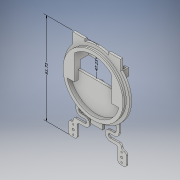
# Autodesk Inventor part: vivetouchpad
Saved by Autodesk Inventor 2019.4 (Build 234330000, 330)
## iProperties
Created: 2021-01-30
Part Number: vivetouchpad
Material: Generic
Document SubType Name: Modeling
Designer: Ian
Density: 1 g/cm^3
Appearance: Default
Author: Ian
Autodesk Inventor part; units mm, degrees
ref_plane "YZ Plane" through (0, 0, 0) normal (1, 0, 0) x (0, 1, 0)
ref_plane "XZ Plane" through (0, 0, 0) normal (0, 1, 0) x (-1, 0, 0)
ref_plane "XY Plane" through (0, 0, 0) normal (0, 0, 1) x (1, 0, 0)
sketch "Sketch1" plane through (0, 0, 0) normal (0, 0, 1) x (1, 0, 0)
  circle A0 centre (0, 0) radius 22
  line L0 (-4, -21.6333) -> (-4, -25.1333)
  line L1 (-4, -25.1333) -> (4, -25.1333)
  line L2 (4, -25.1333) -> (4, -21.6333)
  line L3 (-16, 15.0997) -> (-16, 22.0997)
  line L4 (-16, 22.0997) -> (-8, 22.0997)
  line L5 (-8, 22.0997) -> (-8, 20.4939)
  line L6 (8, 20.4939) -> (8, 22.0997)
  line L7 (8, 22.0997) -> (16, 22.0997)
  line L8 (16, 22.0997) -> (16, 15.0997)
  circle A1 centre (0, 0) radius 2.75
  circle A2 centre (0, 0) radius 1.25 construction
  circle A3 centre (0, 0) radius 1.35
  dimension "d0" = 44
  dimension "d1" = 8
  dimension "d2" = 16
  dimension "d3" = 7
  dimension "d4" = 8
  dimension "d5" = 3.5
  dimension "d6" = 2.5
  dimension "d7" = 0.1
  dimension "d8" = 5.5
  constraints: 18 end point, 6 point on circle, 5 perpendicular, 4 centre point, 4 parallel, 3 coincident, 2 point on line, 2 vertical
  measures "d0" diameter of A0
  measures "d1" distance of L6.end L7.end
  measures "d2" distance between parallel lines of L6 L5
  measures "d3" distance of L7.end L8.end
  measures "d4" distance of L0.end L1.end
  measures "d5" distance of L1.end L2.end
  measures "d6" diameter of A2
  measures "d7" radial gap between concentric circles of A2 A3
  measures "d8" diameter of A1
extrude "Extrusion1" add sketch "Sketch1" along normal blind 1.5 contours A0 | A0 L6 L7 L8 | L2 L1 L0 A0 | A0 L3 L4 L5 | A1 | A3
sketch "Sketch10" plane through (0, 0, 0) normal (0, 0, -1) x (-1, 0, 0)
  circle A0 centre (0, -1.6753) radius 1.25 construction
  circle A1 centre (0, -1.6753) radius 2.625
  line L0 (-16, 22.0997) -> (-8, 22.0997) construction
  point P0 (0, 0)
  dimension "d85" = 5.25
  dimension "d86" = 2.5
  dimension "d87" = 26.4
  constraints: 2 centre point, 1 coincident, 1 vertical alignment
  measures "d85" diameter of A1
  measures "d86" diameter of A0
extrude "Extrusion8" add sketch "Sketch10" along normal blind 2.3
sketch "Sketch11" plane through (0, -1.6753, -2.3) normal (0, 0, -1) x (-1, 0, 0)
  circle A0 centre (0, 0) radius 1.25 construction
  circle A1 centre (0, 0) radius 1.35
  circle A2 centre (0, 0) radius 1.65
  point P0 (0, 1.6753)
  dimension "d90" = 2.5
  dimension "d91" = 0.1
  dimension "d92" = 0.3
  constraints: 3 centre point
  measures "d90" diameter of A0
  measures "d91" radial gap between concentric circles of A0 A1
  measures "d92" radial gap between concentric circles of A1 A2
extrude "Extrusion9" add sketch "Sketch11" along normal blind 0.2
chamfer "Chamfer1" distance 0.975 angle 45 1 edges at (2.625, -1.6753, -2.3)
fillet "Fillet1" radius 2 1 edges at (2.625, -1.6753, -1.3251)
fillet "Fillet2" radius 0.5 2 edges at (1.6501, -1.6753, -2.3) (1.65, -1.6753, -2.3)
sketch "Sketch8" plane through (0, 0, 1.5) normal (0, 0, 1) x (1, 0, 0)
  circle A0 centre (0, 0) radius 1.35 projected
  circle A1 centre (0, 0) radius 19.875
  circle A2 centre (0, 0) radius 17.875
  dimension "d78" = 39.75
  dimension "d79" = 2
  constraints: 2 centre point, 1 coincident
  measures "d78" diameter of A1
  measures "d79" radial gap between concentric circles of A1 A2
extrude "Extrusion6" add sketch "Sketch8" along normal blind 2.5 contours A1
sketch "Sketch9" plane through (0, 0, 4) normal (0, 0, 1) x (1, 0, 0)
  circle A0 centre (0, 0) radius 17.875 projected
  circle A1 centre (0, 0) radius 19.875 projected
  circle A2 centre (0, 0) radius 20.15
  dimension "d82" = 40.3
  constraints: 1 centre point, 1 coincident
  measures "d82" diameter of A2
extrude "Extrusion7" add sketch "Sketch9" against normal blind 1 contours A1 | A2
sketch "Sketch12" plane through (0, 0, 0) normal (0, 0, -1) x (-1, 0, 0)
  line L0 (-12.5, 1.875) -> (12.5, 1.875)
  circle A0 centre (0, 0) radius 17.875 construction
  circle A1 centre (0, -1.6753) radius 2.625 construction
  arc A2 (12.5, 12.7775) -> (-12.5, 12.7775) centre (0, 0) ccw
  line L1 (-12.5, 12.7775) -> (-12.5, 1.875)
  line L2 (12.5, 1.875) -> (12.5, 12.7775)
  dimension "d100" = 25
  dimension "d101" = 16
  dimension "d102" = 6.1753
  constraints: 6 end point, 4 point on circle, 2 concentric, 2 parallel, 1 centre point, 1 horizontal, 1 vertical
  measures "d100" distance of L0.start L0.end
  measures "d101" distance edge to line of A0 L0
extrude "Extrusion10" cut sketch "Sketch12" against normal through all
sketch "Sketch6" plane through (0, 0, 0) normal (0, 0, -1) x (-1, 0, 0)
  arc A0 (8.5, -23.1333) -> (8.5, -29.6333) centre (8.5, -26.3833) ccw
  arc A1 (8.5, -25.1333) -> (8.5, -27.6333) centre (8.5, -26.3833) ccw
  line L0 (4, -25.1333) -> (-4, -25.1333) construction
  line L1 (-4, -25.1333) -> (29.2645, -25.1333) construction
  line L2 (0, -1.6753) -> (0, -71.0097) construction
  line L3 (8.5, -26.3833) -> (8.5, -20.6854) construction
  arc A2 (4, -21.6333) -> (16, 15.0997) centre (0, 0) ccw construction
  line L4 (16, 22.0997) -> (16, 15.0997) projected
  line L5 (8, 22.0997) -> (16, 22.0997) projected
  line L6 (8, 20.4939) -> (8, 22.0997) projected
  arc A3 (8, 20.4939) -> (-8, 20.4939) centre (0, 0) ccw projected
  line L7 (-8, 22.0997) -> (-8, 20.4939) projected
  line L8 (-16, 22.0997) -> (-8, 22.0997) projected
  line L9 (-16, 15.0997) -> (-16, 22.0997) projected
  arc A4 (-16, 15.0997) -> (-4, -21.6333) centre (0, 0) ccw projected
  line L10 (-4, -25.1333) -> (-4, -21.6333) projected
  line L11 (4, -25.1333) -> (-4, -25.1333) projected
  line L12 (4, -21.6333) -> (4, -25.1333) projected
  arc A5 (4, -21.6333) -> (16, 15.0997) centre (0, 0) ccw projected
  line L13 (8.5, -27.6333) -> (14.5, -27.6333)
  line L14 (8.5, -29.6333) -> (12.0333, -29.6333)
  line L15 (19.5, -32.6333) -> (19.5, -37.9666)
  line L16 (17.8333, -39.6333) -> (15.3667, -39.6333)
  line L17 (17.8333, -39.6333) -> (13.7, -39.6333)
  line L18 (13.7, -37.9666) -> (13.7, -32.6333)
  line L19 (13.7, -32.6333) -> (19.5, -32.6333) construction
  line L20 (19.5, -32.6333) -> (19.5, -37.9666)
  circle A6 centre (16.25, -32.1333) radius 0.5
  circle A7 centre (16.25, -38.1333) radius 0.5
  circle A8 centre (16.25, -35.1333) radius 0.75
  line L21 (16.25, -35.1333) -> (16.25, -32.1333) construction
  line L22 (16.25, -35.1333) -> (16.25, -38.1333) construction
  arc A9 (19.5, -32.6333) -> (17.8333, -30.9666) centre (17.8333, -32.6333) ccw
  arc A10 (16.1667, -29.3) -> (17.8333, -30.9666) centre (17.8333, -29.3) ccw
  arc A11 (16.1667, -29.3) -> (14.5, -27.6333) centre (14.5, -29.3) ccw
  arc A12 (13.7, -31.3) -> (12.0333, -29.6333) centre (12.0333, -31.3) ccw
  line L23 (13.7, -32.6333) -> (13.7, -31.3)
  arc A13 (17.8333, -39.6333) -> (19.5, -37.9666) centre (17.8333, -37.9666) ccw
  arc A14 (13.7, -37.9666) -> (15.3667, -39.6333) centre (15.3667, -37.9666) ccw
  arc A15 (4, -21.6333) -> (16, 15.0997) centre (0, 0) ccw projected
  line L24 (16, 22.0997) -> (16, 15.0997) construction
  line L25 (16, 22.0997) -> (16, -20.6854) construction
  line L26 (8.5, -23.1333) -> (11.25, -23.1333)
  line L27 (8.5, -25.1333) -> (11.25, -25.1333)
  circle A16 centre (0, -1.6753) radius 2.625 projected
  arc A17 (11.25, -25.1333) -> (14.5, -21.8833) centre (11.25, -21.8833) ccw
  arc A18 (11.25, -23.1333) -> (12.5, -21.8833) centre (11.25, -21.8833) ccw
  line L28 (14.5, -21.8833) -> (14.5, -16.7705)
  line L29 (12.5, -21.8833) -> (12.5, -19.0329)
  arc A19 (12.5, -18.1039) -> (14.5, -16.5454) centre (0, 0) ccw
  arc A20 (12.5, -19.0329) -> (11.7333, -18.6099) centre (12, -19.0329) ccw
  arc A21 (14.6667, -16.3978) -> (14.5, -16.7705) centre (15, -16.7705) ccw
  arc A22 (11.7333, -18.6099) -> (14.6667, -16.3978) centre (0, 0) ccw
  point P0 (19.5, -39.6333)
  dimension "d45" = 2
  dimension "d46" = 6.5
  dimension "d49" = 5.25
  dimension "d53" = 19.5
  dimension "d54" = 10
  dimension "d55" = 5.8
  dimension "d56" = 7
  dimension "d58" = 2.5
  dimension "d61" = 1
  dimension "d63" = 7
  dimension "d64" = 1
  dimension "d65" = 2.75
  dimension "d66" = 1.5
  dimension "d67" = 1.6667
  dimension "d68" = 1.6667
  dimension "d75" = 22
  dimension "d119" = 2
  dimension "d120" = 1.5
  dimension "d121" = 0.5
  dimension "d122" = 0.5
  constraints: 38 end point, 31 point on circle, 22 tangent, 17 centre point, 10 equal radius, 9 point on line, 8 vertical, 6 horizontal, 2 parallel, 2 vertical alignment, 1 coincident, 1 collinear, 1 concentric, 1 horizontal alignment, 1 perpendicular
  measures "d45" radial gap between concentric circles of A0 A1
  measures "d46" diameter of A0
  measures "d49" distance edge to line of A0 L2
  measures "d53" distance between parallel lines of L2 L15
  measures "d54" distance between parallel lines of L14 L16
  measures "d55" distance of L18.end L15.start
  measures "d56" distance of L17.end L18.end
  measures "d58" diameter of A1
  measures "d61" diameter of A6
  measures "d64" distance edge to line of A7 L17
  measures "d65" distance edge to line of A7 L20
  measures "d66" diameter of A8
  measures "d67" radius of A9
  measures "d68" radius of A13
  measures "d75" radius of A2
  measures "d119" distance between parallel lines of L29 L28
  measures "d120" distance between parallel lines of L25 L28
  measures "d121" radius of A20
  measures "d122" radius of A21
extrude "Extrusion5" add sketch "Sketch6" against normal blind 1 contours L26 A18 L29 A20 A5 A21 L28 A17 L27 A1 L13 A11 A10 A9 L15 A13 L16 A14 L18 L23 A12 L14 A0
mirror "Mirror1" about plane through (0, 0, 0) normal (1, 0, 0) of "Extrusion5"
sketch "Sketch13" plane through (0, 0, 1.5) normal (0, 0, 1) x (1, 0, 0)
  line L0 (-12.5, 12.7775) -> (-12.5, 1.875) projected
  line L1 (-12.5, 12.7775) -> (-12.5, 1.875)
  line L2 (-12.5, 1.875) -> (-12.5, -4.125)
  line L3 (-12.5, -4.125) -> (-17.3925, -4.125)
  arc A0 (-12.5, 12.7775) -> (12.5, 12.7775) centre (0, 0) ccw projected
  line L4 (12.5, 1.875) -> (-12.5, 1.875) projected
  line L5 (12.5, 1.875) -> (12.5, -4.125)
  line L6 (12.5, -4.125) -> (17.3925, -4.125)
  line L7 (12.5, 1.875) -> (12.5, 12.7775) projected
  arc A1 (17.3925, -4.125) -> (12.5, 12.7775) centre (0, 0) ccw
  arc A2 (-12.5, 12.7775) -> (-17.3925, -4.125) centre (0, 0) ccw
  circle A3 centre (0, 0) radius 17.875 projected
  line L8 (12.5, 1.875) -> (12.5, 12.7775)
  line L9 (-12.5, 12.7775) -> (-12.5, -4.125)
  line L10 (12.5, -4.125) -> (12.5, 12.7775)
  dimension "d108" = 6
  constraints: 16 end point, 5 point on circle, 4 concentric, 3 equal length, 3 point on line, 2 centre point, 2 perpendicular, 1 vertical
  measures "d108" distance of L0.end L2.end
extrude "Extrusion11" add sketch "Sketch13" along normal up to surface (2.5 mm away) contours L0 L2 L3 A0 | A0 L6 L5 L7
ref_plane "Work Plane1" through (-16, 11.9873, 0) normal (0, 1, 0) x (1, 0, 0)
sketch "Sketch14" plane through (-16, 11.9873, 0) normal (0, 1, 0) x (1, 0, 0)
  line L0 (3.5, -4) -> (3.5, 0) projected
  line L1 (3.5, 0) -> (3.5, 5.5)
  line L2 (3.5, 5.5) -> (8.5, 5.5)
  line L3 (3.5, 0) -> (2.5, 0)
  line L4 (8, 0) -> (0, 0) projected
  line L5 (2.5, 0) -> (2.5, 6.5)
  line L6 (2.5, 6.5) -> (8.5, 6.5)
  line L7 (8.5, 6.5) -> (8.5, 5.5)
  line L8 (28.5, 0) -> (28.5, -4) projected
  line L9 (28.5, 0) -> (28.5, 5.5)
  line L10 (28.5, 5.5) -> (26.75, 5.5)
  line L11 (26.75, 5.5) -> (26.75, 6.5)
  line L12 (26.75, 6.5) -> (29.5, 6.5)
  line L13 (29.5, 6.5) -> (29.5, 0)
  line L14 (32, 0) -> (24, 0) projected
  line L15 (28.5, 0) -> (29.5, 0)
  point P0 (16, 0)
  dimension "d111" = 1
  dimension "d112" = 6.5
  dimension "d113" = 1
  dimension "d114" = 6
  dimension "d117" = 1
  dimension "d118" = 1.75
  constraints: 24 end point, 6 perpendicular, 3 vertical, 2 collinear, 2 horizontal, 2 point on line
  measures "d111" distance of L0.end L3.end
  measures "d112" distance of L3.end L5.end
  measures "d113" distance between parallel lines of L6 L2
  measures "d114" distance of L5.end L6.end
  measures "d117" distance between parallel lines of L9 L13
  measures "d118" distance of L9.end L10.end
extrude "Extrusion12" add sketch "Sketch14" against normal blind 5
body "Solid1"
